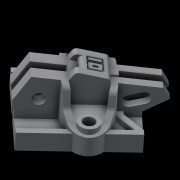
# Autodesk Inventor part: SpineNeckLink
Saved by Autodesk Inventor 2015 (Build 190159000, 159)
## iProperties
Created: 2015-01-12
Part Number: SpineNeckLink
Material: Generic
Document SubType Name: Modeling
Designer: Inventor
Density: 1 g/cm^3
Appearance: Default
Mass: 29.1687 g
Surface Area: 115.943 cm^2
Volume: 29.1687 cm^3
RuleStatus: InUse
BeforeDocSave0: UpdateBoundingBox
CX: 62.74 mm
CY: 47.85 mm
CZ: 29.34 mm
Author: Inventor
Autodesk Inventor part; units mm, degrees
ref_plane "YZ Plane" through (0, 0, 0) normal (1, 0, 0) x (0, 1, 0)
ref_plane "XZ Plane" through (0, 0, 0) normal (0, 1, 0) x (-1, 0, 0)
ref_plane "XY Plane" through (0, 0, 0) normal (0, 0, 1) x (1, 0, 0)
sketch "Body" plane through (0, 0, 0) normal (0, 0, 1) x (1, 0, 0)
  circle A0 centre (0, -17.5) radius 3
  arc A1 (-11.5, -8) -> (-8.4334, -18) centre (26.9827, -1.6692) ccw
  arc A2 (-8.4334, -18) -> (0, -24.0453) centre (1.1017, -13.6032) ccw
  line L0 (0, -24.0453) -> (0, -4) construction
  line L1 (-29, -4) -> (-29, -21)
  line L2 (-29, -21) -> (-6.3507, -21)
  line L3 (-29, -4) -> (0, -4)
  line L4 (-29, -8) -> (0, -8)
  line L5 (-29, -4) -> (-29, 0) construction
  line L6 (-29, 0) -> (0, 0) construction
  line L7 (0, 0) -> (0, -4) construction
  arc A3 (8.4334, -18) -> (11.5, -8) centre (-26.9827, -1.6692) ccw
  arc A4 (0, -24.0453) -> (8.4334, -18) centre (-1.1017, -13.6032) ccw
  line L8 (6.3507, -21) -> (22, -21)
  line L9 (22, -21) -> (22, -8)
  line L10 (0, -8) -> (22, -8)
  line L11 (22, -8) -> (22, -4)
  line L12 (0, -4) -> (22, -4)
  line L13 (22, -4) -> (22, 0) construction
  line L14 (0, 0) -> (22, 0) construction
  line L15 (-29, -18) -> (-8.4334, -18) construction
  line L16 (22, -18) -> (8.4334, -18) construction
  line L17 (-9, -4) -> (-9, 0)
  line L18 (4, -4) -> (4, 0)
  line L19 (-9, 0) -> (4, 0)
  line L20 (18.2436, -18) -> (10.7081, -8) construction
  line L21 (22, -18) -> (14.4645, -8) construction
  line L22 (-9, -4) -> (-9, -2)
  line L23 (-29, -4) -> (-29, -2)
  line L24 (-9, -2) -> (-29, -2)
  line L25 (4, -2) -> (22, -2)
  line L26 (22, -4) -> (22, -2)
  dimension "d0" = 6
  dimension "d1" = 4
  dimension "d2" = 17
  dimension "d3" = 4
  dimension "d4" = 3
  dimension "d5" = 29
  dimension "d6" = 22
  dimension "d7" = 53
  dimension "d8" = 3
  dimension "d9" = 20
  dimension "d10" = 18
  dimension "d11" = 22.6493
  dimension "d14" = 11.5
  dimension "d15" = 10.5
  dimension "d16" = 39
  dimension "d17" = 9.5
  constraints: 54 end point, 13 point on line, 11 point on circle, 8 vertical, 6 horizontal, 6 perpendicular, 5 centre point, 4 midpoint, 4 symmetric about line, 3 collinear, 1 coincident, 1 parallel, 1 tangent, 2 other
  measures "d0" diameter of A0
  measures "d1" distance between parallel lines of L3 L4
  measures "d2" distance of L1.start L1.end
  measures "d3" distance of L1.start L5.end
  measures "d4" distance between parallel lines of L2 L15
  measures "d5" distance of L1.start L0.end
  measures "d6" distance of L0.end L11.end
  measures "d7" angle of L20 L16
  measures "d8" distance between parallel lines of L21 L20
  measures "d9" distance between parallel lines of L1 L17
  measures "d10" distance between parallel lines of L13 L18
  measures "d11" distance of L1.end L2.end
  measures "d14" distance of L4.end A1.start
  measures "d15" radius of A4
  measures "d16" radius of A3
  measures "d17" distance of L4.end A0.centre
extrude "BodyFeature" add sketch "Body" along normal blind 6 contours L4 L10 A3 A4 A2 A1 | A1 A2 L2 L1 L4 | L4 L1 L3 L12 L11 L10 | L10 L9 L8 A4 A3 | L17 L19 L18 L12 L3 | L12 L18 L25 L26
sketch "Mount" plane through (0, 0, 6) normal (0, 0, 1) x (1, 0, 0)
  arc A0 (-6.3507, -21) -> (0, -24.0453) centre (1.1017, -13.6032) ccw projected
  arc A1 (0, -24.0453) -> (6.3507, -21) centre (-1.1017, -13.6032) ccw projected
  arc A2 (-11.5, -8) -> (-8.4334, -18) centre (26.9827, -1.6692) ccw projected
  arc A3 (8.4334, -18) -> (11.5, -8) centre (-26.9827, -1.6692) ccw projected
  line L0 (-11.5, -8) -> (11.5, -8)
  arc A4 (-8.4334, -18) -> (0, -24.0453) centre (1.1017, -13.6032) ccw projected
  arc A5 (0, -24.0453) -> (8.4334, -18) centre (-1.1017, -13.6032) ccw projected
  circle A6 centre (0, -17.5) radius 3 projected
  constraints: 2 end point, 1 horizontal
extrude "MountFeature" add sketch "Mount" along normal blind 7.5
extrude "RidgeFeature" add sketch "Body" along normal blind 27 contours L4 L1 L3 L12 L11 L10 | L23 L24 L17 L3 | L17 L19 L18 L12 L3 | L12 L18 L25 L26
sketch "Borders" plane through (0, 0, 6) normal (0, 0, 1) x (1, 0, 0)
  line L0 (-29, -18) -> (-8.4334, -18) projected
  line L1 (22, -18) -> (8.4334, -18) projected
  line L2 (18.2436, -18) -> (10.7081, -8) projected
  line L3 (22, -18) -> (14.4645, -8) projected
  line L4 (-29, -18) -> (-29, -21)
  line L5 (-29, -21) -> (-6.3507, -21)
  line L6 (-29, -21) -> (-6.3507, -21) projected
  line L7 (-6.3507, -21) -> (-8.4334, -18)
  arc A0 (-8.4334, -18) -> (-6.3507, -21) centre (1.1017, -13.6032) ccw projected
  line L8 (8.4334, -18) -> (6.3507, -21)
  line L9 (6.3507, -21) -> (22, -21)
  line L10 (6.3507, -21) -> (22, -21) projected
  line L11 (22, -21) -> (22, -18)
  line L12 (10.7081, -8) -> (14.4645, -8)
  constraints: 14 end point, 2 collinear, 2 perpendicular, 1 vertical
extrude "BordersFeature" add sketch "Borders" along normal blind 3 contours L0 A0 L5 L4 | L11 L9 L8 L1 | L1 L2 L12 L3
move faces "Move1" translate (20, 0, 0) faces at (22, -4, 11)
move faces "Move2" translate (-20, 0, 0) faces at (-29, -4, 11)
sketch "SideProfile" plane through (-11.5, -8, 13.5) normal (0, -1, 0) x (1, 0, 0)
  line L0 (-37.5, -7.5) -> (-37.5, 13.5) construction
  line L1 (53.5, -7.5) -> (53.5, 13.5) construction
  line L2 (-37.5, -13.5) -> (5.1493, -13.5) construction
  line L3 (33.5, 13.5) -> (33.5, -13.5) construction
  line L4 (-17.5, -13.5) -> (33.5, -13.5)
  line L5 (33.5, -13.5) -> (33.5, -4.5)
  line L6 (17.8507, -4.5) -> (35.7607, -4.5) construction
  line L7 (-17.5, -13.5) -> (-17.5, -4.5)
  line L8 (-17.5, -4.5) -> (-18.7376, 1.5)
  line L9 (-18.7376, 1.5) -> (-11.8094, 13.5)
  line L10 (-11.8094, 13.5) -> (41, 7.5)
  line L11 (41, 7.5) -> (44, 2)
  line L12 (44, 2) -> (33.5, -4.5)
  line L13 (-37.5, -4.5) -> (5.1493, -4.5) construction
  line L14 (-37.5, 13.5) -> (53.5, 13.5) construction
  line L15 (-20.9223, 1.5) -> (-11.6847, 17.5) construction
  line L16 (-19.6847, -4.5) -> (-20.9223, 1.5) construction
  line L17 (-20.9223, 1.5) -> (-18.7376, 1.5) construction
  dimension "d31" = 20
  dimension "d55" = 12
  dimension "d56" = 10.5
  dimension "d62" = 20
  dimension "d68" = 3
  dimension "d69" = 18
  dimension "d91" = 6.5
  constraints: 20 end point, 5 point on line, 2 horizontal, 2 parallel, 1 perpendicular, 1 vertical
  measures "d31" distance between parallel lines of L3 L1
  measures "d55" vertical distance of L5.end L10.end
  measures "d56" distance from line of L11.end L3
  measures "d62" distance between parallel lines of L0 L7
  measures "d68" horizontal distance of L10.end L11.end
  measures "d69" distance from line of L3.start L6
  measures "d91" distance from line of L6 L11.end
extrude "SideProfileFeature" cut sketch "SideProfile" along normal through all both and the other way through all keep common part
sketch "SpineMountHole" plane through (-11.5, -8, 13.5) normal (0, -1, 0) x (1, 0, 0)
  circle A0 centre (-8.1847, 2.5) radius 3.25
  line L0 (-18.7376, 1.5) -> (-11.8094, 13.5) construction
  line L1 (-17.5, -4.5) -> (-18.7376, 1.5) construction
  line L2 (-11.8094, 13.5) -> (41, 7.5) construction
  arc A1 (-9.9054, 0.0425) -> (-6.464, 4.9575) centre (-8.1847, 2.5) ccw projected
  dimension "d35" = 6.5
  constraints: 1 centre point, 1 coincident
  measures "d35" diameter of A0
hole "SpineMountHoleFeature" at (-19.6847, -8, 16) direction (0, 1, 0) diameter 6 end through all
sketch "SpineMountHole2" plane through (-11.5, -8, 13.5) normal (0, -1, 0) x (1, 0, 0)
  circle A0 centre (33.6227, 2.2271) radius 3.25 projected
hole "SpineMountHole2Feature" at (22.1227, -8, 15.7271) direction (0, 1, 0) diameter 6 end through all
fillet "FilletRestoreFeature" radius 7 1 edges at (0, -24.0453, 6.75)
ref_plane "MountSlopePlane" through (11.5, -8, 13.5) normal (0, -0.258819, 0.9659258) x (-1, 0, 0)
sketch "MountSlope" plane through (11.5, -8, 13.5) normal (0, -0.258819, 0.9659258) x (-1, 0, 0)
  line L0 (23.8185, 0) -> (-1.268, 0)
  line L1 (-1.268, 0) -> (-1.268, 17.2999)
  line L2 (-1.268, 17.2999) -> (23.8185, 17.2999)
  line L3 (23.8185, 17.2999) -> (23.8185, 0)
  point P0 (11.5, -4.2333)
  constraints: 8 end point, 2 parallel, 1 horizontal, 1 perpendicular
extrude "MountSlopeFeature" cut sketch "MountSlope" along normal through all
sketch "MountRaise" plane through (0, 0, 9) normal (0, 0, 1) x (1, 0, 0)
  circle A0 centre (0, -17.5) radius 3 projected
  circle A1 centre (0, -17.5) radius 5
  point P0 (0, 0)
  dimension "d73" = 2
  constraints: 1 centre point, 1 coincident
  measures "d73" radial gap between concentric circles of A1 A0
extrude "MountRaiseFeature" add sketch "MountRaise" along normal blind 3.5
sketch "FrontHole" plane through (11.5, -8, 9) normal (0, -1, 0) x (1, 0, 0)
  circle A0 centre (10.6227, 6.7271) radius 3 projected
  line L0 (10.6227, 6.7271) -> (4.8343, 5.148) construction
  circle A1 centre (4.8343, 5.148) radius 3
  line L1 (21, 6.5) -> (10.5, 0) projected
  line L2 (4.0447, 8.0422) -> (9.8332, 9.6213)
  line L3 (5.6238, 2.2537) -> (11.4123, 3.8329)
  dimension "d158" = 6
  dimension "d159" = 6
  dimension "d160" = 16.5
  constraints: 6 end point, 4 point on circle, 3 tangent, 1 centre point, 1 coincident, 1 parallel
  measures "d158" diameter of A1
  measures "d159" distance of L0.start L0.end
  measures "d160" angle of L0 L1
extrude "FrontHoleFeature" cut sketch "FrontHole" against normal through all
sketch "MountRidges" plane through (0, 0, 9) normal (0, 0, 1) x (1, 0, 0)
  arc A0 (-11.5, -8) -> (-8.4334, -18) centre (26.9827, -1.6692) ccw
  arc A1 (-11.5, -8) -> (-8.4334, -18) centre (26.9827, -1.6692) ccw projected
  arc A2 (-8.4334, -18) -> (-6.3507, -21) centre (1.1017, -13.6032) ccw
  arc A3 (-8.4334, -18) -> (-2.2034, -23.5695) centre (1.1017, -13.6032) ccw projected
  line L0 (-6.3507, -21) -> (-5, -17.9644)
  line L1 (11.5, -8) -> (-11.5, -8) projected
  arc A4 (-8.4562, -8) -> (-5.7091, -16.7438) centre (26.9827, -1.6692) ccw
  arc A5 (-5.7091, -16.7438) -> (-5, -17.9644) centre (1.1017, -13.6032) ccw
  line L2 (0, -8) -> (0, -24.1693) construction
  arc A6 (8.4334, -18) -> (11.5, -8) centre (-26.9827, -1.6692) ccw
  line L3 (6.3507, -21) -> (5, -17.9644)
  arc A7 (5.7091, -16.7438) -> (8.4562, -8) centre (-26.9827, -1.6692) ccw
  arc A8 (5, -17.9644) -> (5.7091, -16.7438) centre (-1.1017, -13.6032) ccw
  line L4 (8.4562, -8) -> (11.5, -8)
  arc A9 (6.3507, -21) -> (8.4334, -18) centre (-1.1017, -13.6032) ccw
  arc A10 (2.2034, -23.5695) -> (8.4334, -18) centre (-1.1017, -13.6032) ccw projected
  dimension "d92" = 3
  dimension "d95" = 5
  constraints: 16 point on circle, 8 centre point, 8 end point, 8 symmetric about line, 4 tangent, 2 concentric, 1 collinear, 1 midpoint, 1 point on line, 1 vertical, 3 other
  measures "d95" distance from line of L0.end L2
extrude "MountRidgesFeature" add sketch "MountRidges" along normal up to surface separate body surface through (29.5, -8, 21) normal (0.1128898, 0, 0.9936075)
sketch "MountRidgeProfiles" plane through (-29, -21, 9) normal (-1, 0, 0) x (0, 0, 1)
  line L0 (18, 13) -> (18, 10) construction
  line L1 (18, 10) -> (7.2766, 8.1092)
  arc A0 (7.2766, 8.1092) -> (5.5681, 7.1621) centre (7.7976, 5.1548) ccw
  line L2 (5.5681, 7.1621) -> (1.8205, 3)
  line L3 (1.8205, 3) -> (-0.2077, -4.5695)
  line L4 (18, 10) -> (18, -4.5695)
  line L5 (-0.2077, -4.5695) -> (18, -4.5695)
  line L6 (0.3282, -2.5695) -> (-9, -2.5695) projected
  line L7 (1.8205, 3) -> (0.3282, -2.5695) projected
  dimension "d96" = 3
  dimension "d98" = 3
  dimension "d101" = 2
  dimension "d102" = 80
  dimension "d103" = 142
  constraints: 12 end point, 2 point on circle, 2 tangent, 1 centre point, 1 collinear, 1 horizontal, 1 perpendicular, 1 vertical
  measures "d96" distance of L0.start L0.end
  measures "d98" radius of A0
  measures "d101" distance between parallel lines of L5 L6
  measures "d102" angle of L4 L1
  measures "d103" angle of L1 L2
extrude "MountRidgeProfilesFeature" cut sketch "MountRidgeProfiles" against normal through all bodies 2
combine bodies "MountRidgesJoinFeature" operation type add bodies to combine 2 1
fillet "MountRidgesTopFilletsFeature" radius 3 2 edges at (-9.2618, -11.2814, 25.404) (9.1625, -11.6505, 23.3107)
sketch "CutConnectorRidge" plane through (14.4645, -8, 6) normal (0, -1, 0) x (1, 0, 0)
  line L0 (-2.9645, 3) -> (-2.9645, 17.0451) projected
  line L1 (-2.9645, 3) -> (0, 3) projected
  line L2 (0, 3) -> (0, 0) projected
  line L3 (7.5355, 0) -> (0, 0) projected
  line L4 (7.5355, 3) -> (7.5355, 0) projected
  line L5 (18.0355, 9.5) -> (7.5355, 3) projected
  line L6 (15.0355, 15) -> (18.0355, 9.5) projected
  line L7 (-2.9645, 17.0451) -> (15.0355, 15) projected
  arc A0 (8.4478, 6.8329) -> (6.8687, 12.6213) centre (7.6583, 9.7271) ccw projected
  line L8 (8.4478, 6.8329) -> (2.6594, 5.2537) projected
  arc A1 (1.0802, 11.0422) -> (2.6594, 5.2537) centre (1.8698, 8.148) ccw projected
  line L9 (1.0802, 11.0422) -> (6.8687, 12.6213) projected
  point P0 (-14.4645, -6)
extrude "CutConnectorRidgeFeature" cut sketch "CutConnectorRidge" against normal blind 2 bodies 2
fillet "CutConnectorRidgeFilletFeature" radius 10 1 edges at (11.5, -8, 16.0225)
fillet "MountRidgesTransitionFilletsFeature" radius 5 2 edges at (6.7246, -18, 10.8205) (-6.7246, -18, 10.8205)
mirror "MirrorAllFeature" about plane through (4, 0, 0) normal (0, 1, 0) bodies 2
sketch "Cover" plane through (-8.4562, -8, 13.5) normal (0, -1, 0) x (1, 0, 0)
  line L0 (0, 11.8124) -> (2.8775, 16.099)
  line L1 (2.8775, 16.099) -> (16.9125, 12.8305)
  line L2 (16.9125, 12.8305) -> (16.9125, 9.8909)
  line L3 (0, 11.8124) -> (16.6959, 9.9155)
  line L4 (16.9125, 9.8909) -> (16.6959, 9.9155) projected
  constraints: 8 end point, 1 collinear
extrude "CoverFeature" add sketch "Cover" against normal up to surface (16 mm away) bodies 2
fillet "CoverFilletsFeature" radius 2 2 edges at (-5.5787, 0, 29.599) (8.4562, 0, 26.3305)
ref_plane "MidPlane" through (-8.4562, 0, 13.5) normal (0, -1, 0) x (1, 0, 0)
sketch "CoverCut" plane through (-8.4562, 0, 13.5) normal (0, -1, 0) x (1, 0, 0)
  line L0 (0, 11.8124) -> (2.108, 14.9526) construction
  arc A0 (4.2222, 15.7858) -> (2.108, 14.9526) centre (3.7686, 13.8379) ccw projected
  line L1 (4.2222, 15.7858) -> (15.3661, 13.1906) construction
  line L2 (2.108, 14.9526) -> (0.8941, 13.1444)
  line L3 (0.8941, 13.1444) -> (3.8159, 12.4639)
  line L4 (3.8159, 12.4639) -> (4.5706, 15.7047)
  line L5 (4.5706, 15.7047) -> (4.2222, 15.7858)
  point P0 (8.4562, -13.5)
  dimension "d111" = 1.5
  dimension "d113" = 3
  constraints: 8 end point, 2 point on line, 1 collinear, 1 parallel, 1 perpendicular
  measures "d111" distance from line of L0.start L3
  measures "d113" distance of L2.end L3.end
extrude "CoverCutFeature" cut sketch "CoverCut" along normal mid plane 8 bodies 2
fillet "CoverCutFillet1Feature" radius 2 1 edges at (-3.8856, 0, 29.2047)
fillet "CoverCutFillet2Feature" radius 5 1 edges at (-9, 0, 25.3742)
sketch "MiddleExtend" plane through (4, -2, 0) normal (1, 0, 0) x (0, 0, -1)
  line L0 (-23.8972, 4) -> (-23.8972, 0) projected
  line L1 (0, 0) -> (-23.8972, 0) projected
  line L2 (0, 0) -> (0, 4) projected
  line L3 (0, 4) -> (-23.8972, 4) projected
  point P0 (0, 2)
extrude "MiddleExtendFeature" add sketch "MiddleExtend" along normal blind 8 bodies 2
sketch "Logo" plane through (6.9099, -8, 26.6906) normal (0.2268124, 0, 0.9739385) x (0.9739385, 0, -0.2268124)
  line L0 (-11.4421, 0) -> (0, 0) construction
  line L1 (0, 16) -> (-11.4421, 16) construction
  line L2 (-9.0843, 4) -> (-9.0843, 12) construction
  line L3 (0, 16) -> (0, 0) construction
  line L4 (-0.9797, 4.4375) -> (-0.9797, 12.3125)
  line L5 (-8.1047, 12.3125) -> (-8.1047, 3.6875)
  line L6 (-5.8547, 7.0625) -> (-5.8547, 5.9375)
  line L7 (-5.8547, 5.9375) -> (-3.2297, 5.9375)
  line L8 (-3.2297, 5.9375) -> (-3.2297, 7.0625)
  line L9 (-7.3547, 4.4375) -> (-7.3547, 8.5625)
  line L10 (-1.7297, 4.4375) -> (-1.7297, 3.6875)
  line L11 (-1.7297, 4.4375) -> (-7.3547, 4.4375)
  line L12 (-8.1047, 3.6875) -> (-1.7297, 3.6875)
  line L13 (-3.2297, 7.0625) -> (-5.8547, 7.0625)
  line L14 (-7.3547, 8.5625) -> (-1.7297, 8.5625)
  line L15 (-7.3547, 10.0625) -> (-1.7297, 10.0625)
  line L16 (-7.3547, 11.5625) -> (-7.3547, 10.0625)
  line L17 (-1.7297, 11.5625) -> (-7.3547, 11.5625)
  line L18 (-1.7297, 10.0625) -> (-1.7297, 11.5625)
  line L19 (-0.9797, 12.3125) -> (-8.1047, 12.3125)
  line L20 (-1.7297, 4.4375) -> (-0.9797, 4.4375)
  line L21 (-1.7297, 8.5625) -> (-1.7297, 4.4375)
  dimension "d137" = 8.625
  dimension "d138" = 6.375
  dimension "d139" = 7.125
  dimension "d140" = 0.75
  dimension "d141" = 1.125
  dimension "d142" = 0.75
  dimension "d143" = 0.75
  dimension "d144" = 1.5
  dimension "d145" = 1.5
  dimension "d146" = 0.75
  dimension "d147" = 0.75
  dimension "d148" = 0.75
  dimension "d149" = 1.5
  dimension "d150" = 1.5
  dimension "d151" = 1.5
  dimension "d152" = 3.6875
  dimension "d153" = 3.6875
  dimension "d154" = 0.9797
  dimension "d155" = 0.9797
  constraints: 36 end point, 5 parallel, 3 perpendicular
  measures "d137" distance of L19.end L5.end
  measures "d138" distance of L5.end L10.end
  measures "d139" distance of L19.start L19.end
  measures "d140" distance between parallel lines of L4 L21
  measures "d141" distance between parallel lines of L13 L7
  measures "d142" distance between parallel lines of L19 L17
  measures "d143" distance between parallel lines of L5 L16
  measures "d144" distance between parallel lines of L15 L14
  measures "d145" distance between parallel lines of L9 L6
  measures "d146" distance between parallel lines of L5 L9
  measures "d147" distance between parallel lines of L12 L11
  measures "d148" distance between parallel lines of L4 L18
  measures "d149" distance between parallel lines of L21 L8
  measures "d150" distance between parallel lines of L11 L7
  measures "d151" distance between parallel lines of L14 L13
  measures "d152" distance between parallel lines of L0 L12
  measures "d153" distance between parallel lines of L1 L19
  measures "d154" distance between parallel lines of L2 L5
  measures "d155" distance between parallel lines of L3 L4
extrude "LogoFeature" cut sketch "Logo" against normal blind 2 bodies 2
equation "\"d8\" = d4"
body "Solid2"
